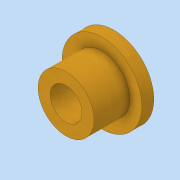
# Autodesk Inventor part: SleeveBearing3mmFlanged
Saved by Autodesk Inventor 2017 (Build 210142000, 142)
## iProperties
Created: 2016-10-06
Part Number: SleeveBearing3mmFlanged
Material: Brass, Soft Yellow, Welded
Document SubType Name: Modeling
Designer: techn
Density: 8.5 g/cm^3
Appearance: Weld - Brass
Author: techn
Autodesk Inventor part; units mm, degrees
ref_plane "YZ Plane" through (0, 0, 0) normal (1, 0, 0) x (0, 1, 0)
ref_plane "XZ Plane" through (0, 0, 0) normal (0, 1, 0) x (-1, 0, 0)
ref_plane "XY Plane" through (0, 0, 0) normal (0, 0, 1) x (1, 0, 0)
sketch "Sketch4" plane through (0, 0, 0) normal (0, 1, 0) x (-1, 0, 0)
  line L0 (2, 0) -> (3.5, 0)
  line L1 (3.5, 0) -> (3.5, 4.5)
  line L2 (3.5, 4.5) -> (2, 4.5)
  line L3 (2, 4.5) -> (2, 0)
  line L4 (2, 0) -> (5, 0)
  line L5 (5, 0) -> (5, -1.5)
  line L6 (5, -1.5) -> (2, -1.5)
  line L7 (2, -1.5) -> (2, 0)
  line L8 (0, -1.5) -> (0, 3.9263)
  point P0 (0, 0)
  dimension "d1" = 1.5
  dimension "d2" = 4.5
  dimension "d3" = 3
  dimension "d4" = 1.5
  dimension "d5" = 4
  constraints: 18 end point, 4 parallel, 2 horizontal, 2 perpendicular, 1 point on line, 1 vertical
  measures "d1" distance of L2.end L1.end
  measures "d2" distance of L1.end L0.end
  measures "d3" distance of L5.end L6.end
  measures "d4" distance of L4.end L5.end
  measures "d5" diameter of L3 L8
revolve "Revolution1" add sketch "Sketch4" angle 360 about axis through (0, 0, -1.5) along (0, 0, 1)
body "Solid1"
